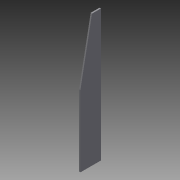
# Autodesk Inventor part: la_side
Saved by Autodesk Inventor 2015 (Build 190159000, 159)
## iProperties
Created: 2015-02-03
Part Number: la_side
Material: Generic
Document SubType Name: Modeling
Designer: rubidium
Density: 1 g/cm^3
Appearance: Default
Author: rubidium
Autodesk Inventor part; units mm, degrees
ref_plane "YZ Plane" through (0, 0, 0) normal (1, 0, 0) x (0, 1, 0)
ref_plane "XZ Plane" through (0, 0, 0) normal (0, 1, 0) x (-1, 0, 0)
ref_plane "XY Plane" through (0, 0, 0) normal (0, 0, 1) x (1, 0, 0)
sketch "Sketch1" plane through (0, 0, 0) normal (1, 0, 0) x (0, 1, 0)
  line L0 (0, -38.1) -> (0, -292.1)
  line L1 (0, -292.1) -> (1879.6, -292.1)
  line L2 (0, -38.1) -> (0, 0)
  line L3 (0, 0) -> (1016, 0)
  line L4 (1016, 0) -> (1879.6, -165.1)
  line L5 (1879.6, -165.1) -> (1879.6, -292.1)
  dimension "d0" = 254
  dimension "d1" = 1879.6
  dimension "d2" = 38.1
  dimension "d3" = 1016
  dimension "d8" = 127
  constraints: 12 end point, 3 perpendicular, 2 vertical, 1 coincident
  measures "d0" distance of L0.start L0.end
  measures "d1" distance of L0.end L1.end
  measures "d2" distance of L0.start L2.end
  measures "d3" distance of L2.end L3.end
  measures "d8" distance of L4.end L1.end
extrude "Extrusion1" add sketch "Sketch1" along normal blind 19.05
body "Solid1"
